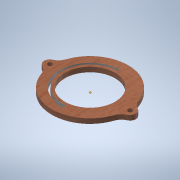
# Autodesk Inventor part: Tussenplaat bevestiging axiale lager
Saved by Autodesk Inventor 2021 (Build 250183000, 183)
## iProperties
Manager: Pierloot J.
Company: Emmaüs Bovenbouw Aalter
Created: 2015-08-18
Part Number: Tussenplaat bevestiging axiale lager
Material: S235
Catalog Web Link: http://emmausbovenbouw.op-weg.be/
Vendor: Emmaüsinstituut Bovenbouw Aalter
Document SubType Name: Modeling
Designer: Pierlootj
Engineer: Pierloot J.
Manufacturer: Standard
Standards Organization: Custom
Density: 7.86 g/cm^3
Appearance: Steel
Title: Algemene titel
Subject: Specifieke titel
Author: Pierlootj
Keywords: Ruwe Ø xxxxx
Comments: Opmerking
Autodesk Inventor part; units mm, degrees
ref_plane "YZ Plane" through (0, 0, 0) normal (1, 0, 0) x (0, 1, 0)
ref_plane "XZ Plane" through (0, 0, 0) normal (0, 1, 0) x (-1, 0, 0)
ref_plane "XY Plane" through (0, 0, 0) normal (0, 0, 1) x (1, 0, 0)
sketch "Sketch1" plane through (0, 0, 0) normal (0, 0, 1) x (1, 0, 0)
  line L0 (0, 2.8582) -> (0, -2.8582) construction
  line L1 (-5.7775, 0) -> (5.7775, 0) construction
  circle A0 centre (0, 0) radius 26.3
  circle A1 centre (0, 0) radius 40
  line L2 (-40, 0) -> (-35, 0)
  circle A2 centre (-35, 0) radius 2.5
  line L3 (40, 0) -> (35, 0)
  circle A3 centre (35, 0) radius 2.5
  dimension "d0" = 52.6
  dimension "d1" = 80
  dimension "d4" = 5
  dimension "d5" = 5
  dimension "d6" = 5
  dimension "d7" = 5
  constraints: 8 end point, 5 coincident, 4 centre point, 3 horizontal, 2 midpoint, 2 point on circle, 1 vertical
  measures "d0" diameter of A0
  measures "d1" diameter of A1
  measures "d4" distance of L2.start L2.end
  measures "d5" diameter of A2
  measures "d6" distance of L3.start L3.end
  measures "d7" diameter of A3
extrude "Extrusion1" add sketch "Sketch1" along normal blind 5 contours A1 | A2 | A3
sketch "Sketch4" plane through (0, 0, 0) normal (0, 0, -1) x (-1, 0, 0)
  line L0 (0, 0) -> (-42, 0)
  line L1 (-42, 0) -> (42, 0)
  circle A0 centre (-42, 0) radius 2.5
  circle A1 centre (-42, 0) radius 6
  circle A2 centre (42, 0) radius 2.5
  circle A3 centre (42, 0) radius 6
  dimension "d19" = 42
  dimension "d20" = 84
  dimension "d21" = 5
  dimension "d22" = 12
  dimension "d23" = 5
  dimension "d24" = 12
  constraints: 4 centre point, 4 coincident, 4 end point, 1 horizontal, 1 point on line
  measures "d19" distance of L0.start L0.end
  measures "d20" distance of L0.end L1.end
  measures "d21" diameter of A0
  measures "d22" diameter of A1
  measures "d23" diameter of A2
  measures "d24" diameter of A3
extrude "Extrusion5" add sketch "Sketch4" against normal blind 5 contours A0 | A1 | A2 | A3
fillet "Fillet2" radius 12 4 edges at (39.619, -5.5074, 2.5) (39.619, 5.5074, 2.5) (-39.619, 5.5074, 2.5) (-39.619, -5.5074, 2.5)
extrude "Extrusion6" cut sketch "Sketch4" against normal blind 5 contours A0 | A2
sketch "Sketch5" plane through (0, 0, 5) normal (0, 0, 1) x (1, 0, 0)
  arc A0 (0, 29.3) -> (0, -29.3) centre (0, 0) ccw
  arc A1 (0, 31.3) -> (-4.25, -31.0101) centre (0, 0) ccw
  line L0 (0, 31.3) -> (0, 29.3)
  line L1 (0, -29.3) -> (4.25, -29.3)
  line L2 (4.25, -29.3) -> (4.25, -32.8)
  line L3 (4.25, -32.8) -> (-4.25, -32.8)
  line L4 (-4.25, -32.8) -> (-4.25, -31.0101)
  dimension "d30" = 29.3
  dimension "d31" = 31.3
  dimension "d32" = 4.25
  dimension "d33" = 3.5
  dimension "d34" = 8.5
  constraints: 10 end point, 4 point on circle, 3 perpendicular, 2 centre point, 2 coincident, 2 vertical
  measures "d30" radius of A0
  measures "d31" radius of A1
  measures "d32" distance of L1.start L1.end
  measures "d33" distance of L1.end L2.end
  measures "d34" distance of L2.end L3.end
extrude "Extrusion7" cut sketch "Sketch5" against normal blind 10
body "Solid1"
